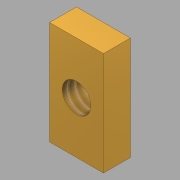
# Autodesk Inventor part: Nut
Saved by Autodesk Inventor 2020 (Build 240168000, 168)
## iProperties
Created: 2019-11-25
Part Number: Nut
Material: Latón, amarillo claro
Document SubType Name: Modeling
Designer: gerar
Density: 8.47 g/cm^3
Appearance: Latón - Satinado
Author: gerar
Autodesk Inventor part; units mm, degrees
ref_plane "YZ Plane" through (0, 0, 0) normal (1, 0, 0) x (0, 1, 0)
ref_plane "XZ Plane" through (0, 0, 0) normal (0, 1, 0) x (-1, 0, 0)
ref_plane "XY Plane" through (0, 0, 0) normal (0, 0, 1) x (1, 0, 0)
sketch "Boceto1" plane through (0, 0, 0) normal (0, 0, 1) x (1, 0, 0)
  line L0 (0, 0) -> (-3.175, 0)
  line L1 (-3.175, 0) -> (-3.175, 6.1034)
  line L2 (-3.175, 6.1034) -> (0, 6.1034)
  line L3 (0, 6.1034) -> (0, 0)
  dimension "d0" = 3.175
  dimension "d1" = 6.1034
  constraints: 8 end point, 2 parallel, 1 horizontal, 1 perpendicular
  measures "d0" distance of L1.end L2.end
  measures "d1" distance between parallel lines of L0 L2
extrude "Extrusión1" add sketch "Boceto1" along normal blind 1.5875
sketch "Boceto2" plane through (0, 0, 1.5875) normal (0, 0, 1) x (1, 0, 0)
  line L0 (-3.175, 0) -> (0, 0) projected
  line L1 (0, 6.1034) -> (-3.175, 6.1034) projected
  line L2 (-3.175, 6.1034) -> (-3.175, 0) projected
  line L3 (0, 0) -> (0, 6.1034) projected
  point P0 (-1.5875, 3.0517)
  dimension "d4" = 6.1034
  dimension "d5" = 3.175
  dimension "d6" = 1.5875
  dimension "d7" = 3.0517
  measures "d4" distance between parallel lines of L0 L1
  measures "d5" distance between parallel lines of L2 L3
  measures "d6" distance from line of L3 point (-1.587, 3.052)
  measures "d7" distance from line of L1 point (-1.587, 3.052)
hole "Agujero1" at (-1.5875, 3.0517, 1.5875) direction (0, 0, -1) diameter 1.6942 end through all thread size "2-56 UNC" class "2B" standard "ANSI Unified Screw Threads"
equation "\"d6\" = 0.5 * d5"
equation "\"d7\" = 0.5 * d4"
